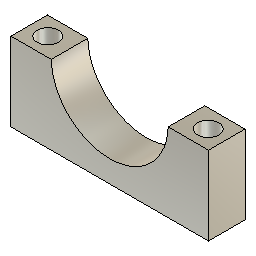
20021-006_arm-clamp (Autodesk Fusion 360 design; units mm, degrees)
Autodesk Fusion 360 part; units mm, degrees
sketch "Sketch1" plane through (0, 0, 0) normal (0, 1, 0) x (1, 0, 0)
  circle A0 centre (0, 0) radius 8
  line L0 (-7.9964, 0.24) -> (-13.51, 0.24)
  line L1 (-13.51, 0.24) -> (-13.51, 11)
  line L2 (-13.51, 11) -> (13.51, 11)
  line L3 (13.51, 11) -> (13.51, 0.24)
  line L4 (13.51, 0.24) -> (7.9964, 0.24)
  point P0 (0, 8)
  dimension "d1" = 27.02
  dimension "d2" = 10.76
  dimension "d3" = 16
  dimension "d4" = 3
  constraint coincident A0.centre origin
  constraint coincident A0 L0.start
  constraint horizontal L0
  constraint perpendicular L0 L1
  constraint perpendicular L1 L2
  constraint perpendicular L2 L3
  constraint coincident A0 L4.end
  constraint perpendicular L3 L4
  constraint equal L0 L4
  constraint equal L1 L3
  constraint coincident A0 P0
  constraint vertical A0.centre P0
  measures "d1" distance of L1 L3
  measures "d2" distance of L2 L4
  measures "d3" diameter of A0
  measures "d4" distance of L2 P0
extrude "Extrude1" add sketch "Sketch1" along normal blind 5 contours A0 L0 L1 L2 L3 L4
sketch "Sketch2" plane through (0, 0, -11) normal (0, 0, -1) x (1, 0, 0)
  line L0 (13.51, 0) -> (-13.51, 0)
  line L1 (-13.51, 0) -> (-13.51, -5)
  line L2 (-13.51, -5) -> (13.51, -5)
  line L3 (13.51, -5) -> (13.51, 0)
  line L4 (-10.97, -2.5) -> (10.97, -2.5) construction
  point P0 (13.51, -2.5)
  point P1 (0, -2.5)
  dimension "d7" = 21.94
  constraint midpoint L3 P0
  constraint parallel L0 L4
  constraint midpoint L4 P1
  constraint vertical origin P1
  constraint horizontal P0 P1
  measures "d7" distance of L4.start L4.end
hole "Hole1" at (-10.97, 2.5, -11) at (10.97, 2.5, -11) direction (0, 0, 1) diameter 2.9 end through all
